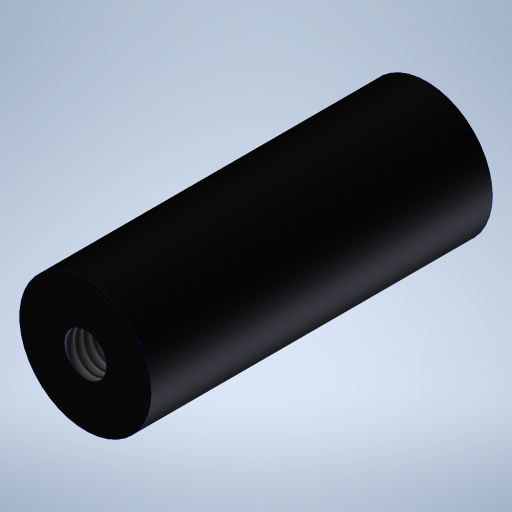
# Autodesk Inventor part: standoff
Saved by Autodesk Inventor 2024 (Build 280153000, 153)
## iProperties
Created: 2024-12-21
Part Number: standoff
Material: Aluminum 6061
Document SubType Name: Modeling
Designer: Danielle
Density: 2.7 g/cm^3
Appearance: Aluminum - Flat
Author: Danielle
Autodesk Inventor part; units mm, degrees
ref_plane "YZ Plane" through (0, 0, 0) normal (1, 0, 0) x (0, 1, 0)
ref_plane "XZ Plane" through (0, 0, 0) normal (0, 1, 0) x (-1, 0, 0)
ref_plane "XY Plane" through (0, 0, 0) normal (0, 0, 1) x (1, 0, 0)
sketch "Sketch1" plane through (0, 0, 0) normal (0, 0, 1) x (1, 0, 0)
  circle A0 centre (0, 0) radius 2.0193
  circle A1 centre (0, 0) radius 6.35
  dimension "d0" = 4.0386
  dimension "d1" = 12.7
  constraints: 2 centre point, 2 coincident
  measures "d0" diameter of A0
  measures "d1" diameter of A1
extrude "Extrusion1" add sketch "Sketch1" along normal blind 32.8422
thread "Thread1" size "8-32 UNC" class "2B" standard "ANSI Unified Screw Threads" full length
body "Solid1"
